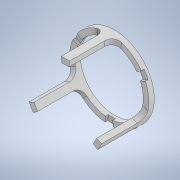
# Autodesk Inventor part: protorheology holder
Saved by Autodesk Inventor 2020.5 (Build 245400000, 400)
## iProperties
Created: 2024-12-03
Part Number: protorheology holder
Material: Generic
Document SubType Name: Modeling
Designer: BassetDC
Density: 1 g/cm^3
Appearance: Default
Author: BassetDC
## iProperties of the stored document _3DPrint.ipt
Created: 2024-12-03
Part Number: _3DPrint
Material: Generic
Document SubType Name: Modeling
Designer: BassetDC
Density: 1 g/cm^3
Appearance: Default
Author: BassetDC
Autodesk Inventor part; units mm, degrees
ref_plane "YZ Plane" through (0, 0, 0) normal (1, 0, 0) x (0, 1, 0)
ref_plane "XZ Plane" through (0, 0, 0) normal (0, 1, 0) x (-1, 0, 0)
ref_plane "XY Plane" through (0, 0, 0) normal (0, 0, 1) x (1, 0, 0)
sketch "Sketch1" plane through (0, 0, 0) normal (0, 0, 1) x (1, 0, 0)
  circle A0 centre (0, 0) radius 12.5
  circle A1 centre (0, 0) radius 14.5
  dimension "d0" = 25
  dimension "d1" = 2
  constraints: 2 centre point, 1 coincident
  measures "d0" diameter of A0
  measures "d1" radial gap between concentric circles of A0 A1
extrude "Extrusion1" add sketch "Sketch1" along normal blind 2
sketch "Sketch2" plane through (0, 0, 2) normal (0, 0, 1) x (1, 0, 0)
  circle A0 centre (0, 0) radius 14.5 construction
  line L0 (0, 14.5) -> (0, 0) construction
  line L1 (0, 0) -> (12.5574, -7.25) construction
  line L2 (0, 0) -> (-12.5574, -7.25) construction
  line L3 (0, 0) -> (-12.5574, 7.25) construction
  line L4 (0, 0) -> (12.5574, 7.25) construction
  circle A1 centre (0, 0) radius 14.5 projected
  circle A2 centre (0, 0) radius 12.5 projected
  line L5 (1.3066, 12.4315) -> (1.5157, 14.4206)
  line L6 (-1.3066, 12.4315) -> (-1.5157, 14.4206)
  line L7 (-11.4193, -5.0842) -> (-13.2464, -5.8977)
  line L8 (-10.1127, -7.3473) -> (-11.7307, -8.5229)
  line L9 (10.1127, -7.3473) -> (11.7307, -8.5229)
  line L10 (11.4193, -5.0842) -> (13.2464, -5.8977)
  line L11 (10.1127, 7.3473) -> (11.7307, 8.5229)
  line L12 (11.4193, 5.0842) -> (13.2464, 5.8977)
  line L13 (-11.4193, 5.0842) -> (-13.2464, 5.8977)
  line L14 (-10.1127, 7.3473) -> (-11.7307, 8.5229)
  line L15 (1.3066, -12.4315) -> (1.5157, -14.4206)
  line L16 (-1.3066, -12.4315) -> (-1.5157, -14.4206)
  point P0 (-12.5574, -7.25)
  point P1 (12.5574, -7.25)
  dimension "d4" = 120
  dimension "d5" = 120
  dimension "d6" = 6
  dimension "d7" = 6
  dimension "d10" = 360
  dimension "d14" = 6
  dimension "d15" = 6
  dimension "d18" = 360
  constraints: 34 end point, 9 point on circle, 1 vertical, 47 other
  measures "d4" angle of L1 L0
  measures "d5" angle of L2 L1
  measures "d6" angle of L0 L6
  measures "d7" angle of L5 L0
  measures "d14" angle of L11 L4
  measures "d15" angle of L12 L4
extrude "Extrusion2" add sketch "Sketch2" along normal blind 16 contours A1 L9 A2 L10 | L5 A2 L6 A1 | A1 L7 A2 L8
sketch "Sketch3" plane through (0, 0, 2) normal (0, 0, 1) x (1, 0, 0)
  circle A0 centre (0, 0) radius 14.5 construction
  line L0 (0, 14.5) -> (0, 0) construction
  line L1 (0, 0) -> (12.5574, -7.25) construction
  line L2 (0, 0) -> (-12.5574, -7.25) construction
  line L3 (0, 0) -> (-12.5574, 7.25) construction
  line L4 (0, 0) -> (12.5574, 7.25) construction
  circle A1 centre (0, 0) radius 14.5
  circle A2 centre (0, 0) radius 12.5
  line L5 (1.3066, 12.4315) -> (1.5157, 14.4206)
  line L6 (-1.3066, 12.4315) -> (-1.5157, 14.4206)
  line L7 (-11.4193, -5.0842) -> (-13.2464, -5.8977)
  line L8 (-10.1127, -7.3473) -> (-11.7307, -8.5229)
  line L9 (10.1127, -7.3473) -> (11.7307, -8.5229)
  line L10 (11.4193, -5.0842) -> (13.2464, -5.8977)
  line L11 (10.1127, 7.3473) -> (11.7307, 8.5229)
  line L12 (11.4193, 5.0842) -> (13.2464, 5.8977)
  line L13 (-11.4193, 5.0842) -> (-13.2464, 5.8977)
  line L14 (-10.1127, 7.3473) -> (-11.7307, 8.5229)
  line L15 (1.3066, -12.4315) -> (1.5157, -14.4206)
  line L16 (-1.3066, -12.4315) -> (-1.5157, -14.4206)
  point P0 (-12.5574, -7.25)
  point P1 (12.5574, -7.25)
  dimension "d24" = 120
  dimension "d25" = 120
  dimension "d26" = 6
  dimension "d27" = 6
  dimension "d28" = 360
  dimension "d29" = 6
  dimension "d30" = 6
  dimension "d31" = 360
  constraints: 34 end point, 9 point on circle, 2 centre point, 1 vertical, 48 other
  measures "d24" angle of L1 L0
  measures "d25" angle of L2 L1
  measures "d26" angle of L0 L6
  measures "d27" angle of L5 L0
  measures "d29" angle of L11 L4
  measures "d30" angle of L12 L4
extrude "Extrusion3" cut sketch "Sketch3" against normal blind 1 contours L12 A2 L11 A1 | A1 L16 A2 L15 | L14 A2 L13 A1
fillet "Fillet1" radius 3 6 edges at (1.4111, 13.426, 2) (-1.4111, 13.426, 2) (-12.3329, -5.4909, 2) (12.3329, -5.4909, 2) (-10.9217, -7.9351, 2) (10.9217, -7.9351, 2)
body "Solid1"
